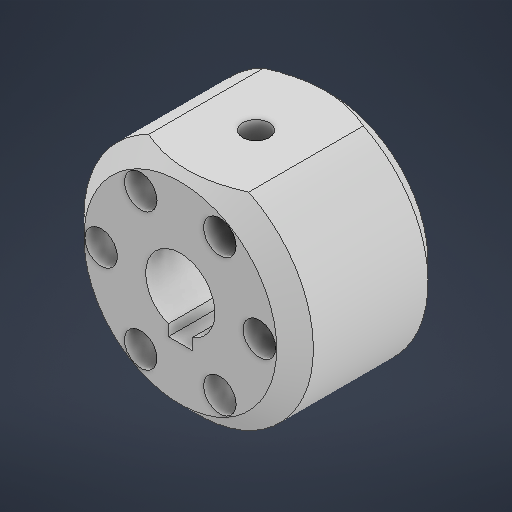
# Autodesk Inventor part: spool_center
Saved by Autodesk Inventor 2026.1 (Build 301233000, 233)
## iProperties
Created: 2023-11-23
Part Number: spool_center
Material: Generic
Document SubType Name: Modeling
Designer: aaron
Density: 1 g/cm^3
Appearance: Default
Author: aaron
Autodesk Inventor part; units mm, degrees
ref_plane "YZ Plane" through (0, 0, 0) normal (1, 0, 0) x (0, 1, 0)
ref_plane "XZ Plane" through (0, 0, 0) normal (0, 1, 0) x (-1, 0, 0)
sketch "Sketch2" plane through (0, 0, 0) normal (0, 0, 1) x (1, 0, 0)
  circle A0 centre (0, 0) radius 25
  line L0 (-17.0079, 22.5) -> (27.1684, 22.5)
  point P0 (10.8972, 22.5)
  point P1 (-10.8972, 22.5)
  dimension "d4" = 50
  dimension "d5" = 22.5
  constraints: 2 end point, 1 centre point, 1 coincident, 1 horizontal
  measures "d4" diameter of A0
  measures "d5" distance from line of L0 A0.centre
extrude "Extrusion2" add sketch "Sketch2" along normal blind 33 contours A0 L0 picked at (1.1654, 4.7055)
sketch "Sketch3" plane through (-10.8972, 22.5, 0) normal (0, 1, 0) x (1, 0, 0)
  circle A0 centre (10.8972, -16.5) radius 2.875
  line L0 (0, 0) -> (0, -33) projected
  line L1 (21.7945, 0) -> (21.7945, -33) projected
  line L2 (21.7945, 0) -> (0, 0) projected
  point P0 (10.8972, 0)
  dimension "d8" = 5.75
  dimension "d9" = 10.8972
  dimension "d10" = 21.7945
  dimension "d11" = 33
  dimension "d12" = 16.5
  constraints: 1 centre point
  measures "d8" diameter of A0
  measures "d9" distance from line of L0 A0.centre
  measures "d10" distance between parallel lines of L0 L1
  measures "d11" distance of L1.start L1.end
  measures "d12" distance from line of L2 A0.centre
extrude "Extrusion3" cut sketch "Sketch3" against normal blind 15
sketch "Sketch11" plane through (0, 0, 33) normal (0, 0, 1) x (1, 0, 0)
  arc A0 (-10.8972, 22.5) -> (10.8972, 22.5) centre (0, 0) ccw projected
  circle A1 centre (0, 0) radius 17.25
  line L0 (-2.6, -9.53) -> (-2.6, -7.0349)
  arc A2 (2.6, -7.0349) -> (-2.6, -7.0349) centre (0, 0) ccw
  line L1 (2.6, -7.0349) -> (2.6, -9.53)
  line L2 (2.6, -9.53) -> (-2.6, -9.53)
  circle A3 centre (0, 0) radius 7.55
  point P0 (15.4196, -3.8129)
  point P1 (2.6, -7.0882)
  point P2 (-2.6, -7.0882)
  dimension "d54" = 34.5
  dimension "d55" = 7.5
  dimension "d56" = 2.4951
  dimension "d57" = 5.2
  dimension "d58" = 9.53
  dimension "d59" = 90
  dimension "d60" = 90
  dimension "d89" = 15.1
  constraints: 6 end point, 3 centre point, 2 coincident, 2 point on circle
  measures "d54" diameter of A1
  measures "d55" radius of A2
  measures "d56" distance of L1.start L1.end
  measures "d57" distance of L1.end L0.start
  measures "d58" distance from line of A2.centre L2
  measures "d59" angle of L2 L0
  measures "d60" angle of L2 L1
  measures "d89" diameter of A3
extrude "Extrusion9" cut sketch "Sketch11" against normal through all contours L0 A3 L1 L2 | A3 L1 A2 L0 | L0 A2 L1 A3
sketch "Sketch13" plane through (0, 0, 33) normal (0, 0, 1) x (1, 0, 0)
  circle A0 centre (0, 0) radius 21
  arc A1 (2.6, -7.0349) -> (-2.6, -7.0349) centre (0, 0) ccw projected
  circle A2 centre (0, 0) radius 26.9677
  dimension "d73" = 42
  constraints: 2 centre point, 2 coincident
  measures "d73" diameter of A0
extrude "Extrusion11" cut sketch "Sketch13" against normal blind 3
sketch "Sketch14" plane through (0, 0, 0) normal (0, 0, -1) x (-1, 0, 0)
  line L0 (2.6, -9.53) -> (-2.6, -9.53) projected
  line L1 (-2.6, -9.53) -> (-2.6, -7.0882) projected
  line L2 (2.6, -7.0882) -> (2.6, -9.53) projected
  arc A0 (-10.8972, 22.5) -> (10.8972, 22.5) centre (0, 0) ccw projected
  line L3 (-10.8972, 22.5) -> (10.8972, 22.5) projected
  circle A1 centre (0, 0) radius 21 projected
  arc A2 (2.6, -7.0882) -> (-2.6, -7.0882) centre (0, 0) ccw projected
  point P0 (4.7697, 22.5)
  point P1 (-4.7697, 22.5)
  constraints: 1 other
extrude "Extrusion12" cut sketch "Sketch14" against normal blind 3 contours L3 A0
sketch "Sketch15" plane through (0, 0, 33) normal (0, 0, 1) x (1, 0, 0)
  circle A0 centre (0, 0) radius 17.25
  line L0 (0, 0) -> (-15.1779, 26.289)
  line L1 (0, 0) -> (0, 30.3502)
  circle A1 centre (-8.625, 14.9389) radius 3.55
  circle A2 centre (-17.25, 0) radius 3.55
  circle A3 centre (-8.625, -14.9389) radius 3.55
  circle A4 centre (8.625, -14.9389) radius 3.55
  circle A5 centre (17.25, 0) radius 3.55
  circle A6 centre (8.625, 14.9389) radius 3.55
  line L2 (0, 0) -> (8.625, 14.9389)
  dimension "d78" = 34.5
  dimension "d80" = 30
  dimension "d81" = 7.1
  dimension "d84" = 360
  dimension "d88" = 30
  constraints: 6 centre point, 6 end point, 1 coincident, 1 point on line, 1 vertical, 16 other
  measures "d80" angle of L0 L1
  measures "d81" diameter of A1
  measures "d88" angle of L2 L1
extrude "Extrusion13" cut sketch "Sketch15" against normal through all contours A0 A5 | A0 A5 | A6 L2 A0 | A0 A6 | A4 A0 | A0 A4 | L2 A6 A0 | A3 A0 | A0 A3 | A1 A0 L0 | L0 A0 A1 | A0 L0 A1 | A0 A1 L0 | A2 A0 | A0 A2
sketch "Sketch16" plane through (-2.6, -9.53, 33) normal (0, 1, 0) x (1, 0, 0)
  circle A0 centre (2.6, 16.5) radius 2.875 projected
  circle A1 centre (2.6, 16.5) radius 3.3
  point P0 (2.6, 33)
  dimension "d90" = 6.6
  constraints: 1 centre point, 1 coincident
  measures "d90" diameter of A1
extrude "Extrusion14" cut sketch "Sketch16" against normal through all contours A0 | A1
ref_plane "Work Plane1" through (0, 0, 16.5) normal (0, 0, -1) x (-1, 0, 0)
sketch "Sketch17" plane through (0, 0, 16.5) normal (0, 0, -1) x (-1, 0, 0)
  circle A0 centre (8.625, -14.9389) radius 3.55 projected
  circle A1 centre (-8.625, -14.9389) radius 3.55 projected
  circle A2 centre (-17.25, 0) radius 3.55 projected
  circle A3 centre (-8.625, 14.9389) radius 3.55 projected
  circle A4 centre (8.625, 14.9389) radius 3.55 projected
  circle A5 centre (17.25, 0) radius 3.55 projected
  point P0 (0, 0)
extrude "Extrusion15" add sketch "Sketch17" along normal mid plane 14
chamfer "Chamfer5" distance 3 angle 45 12 edges at (-12.175, -14.9389, 9.5) (5.075, -14.9389, 9.5) (13.7, 0, 9.5) (5.075, 14.9389, 9.5) (-12.175, 14.9389, 9.5) (-20.8, 0, 9.5) (5.075, -14.9389, 23.5) (13.7, 0, 23.5) (5.075, 14.9389, 23.5) (-12.175, 14.9389, 23.5) (-20.8, 0, 23.5) (-12.175, -14.9389, 23.5)
chamfer "Chamfer6" distance 3 angle 45 2 edges at (-21, 0, 30) (21, 0, 3)
chamfer "Chamfer7" distance 1 angle 45 2 edges at (0, -25, 3) (0, -25, 30)
equation "\"d9\" = 0.5 * d10"
equation "\"d12\" = 0.5 * d11"
body "Solid2"
